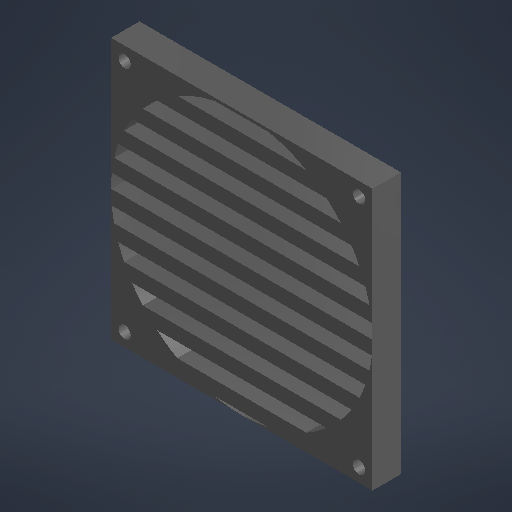
# Autodesk Inventor part: PlaqueProtectionVentilo
Saved by Autodesk Inventor 2026.2 (Build 302298010, 298A)
## iProperties
Part Number: PlaqueProtectionVentilo
Material: Générique
Document SubType Name: Modélisation
Designer: quent
Appearance: Par défaut
Author: quent
Autodesk Inventor part; units mm, degrees
ref_plane "Plan YZ" through (0, 0, 0) normal (1, 0, 0) x (0, 1, 0)
ref_plane "Plan XZ" through (0, 0, 0) normal (0, 1, 0) x (-1, 0, 0)
ref_plane "Plan XY" through (0, 0, 0) normal (0, 0, 1) x (1, 0, 0)
sketch "Esquisse1" plane through (0, 0, 0) normal (0, 0, 1) x (1, 0, 0)
  line L0 (-45.1239, -31.1354) -> (-45.1239, 20.8646)
  circle A0 centre (-40.3739, -46.3854) radius 2.2
  circle A1 centre (-40.3739, 36.1146) radius 2.2
  line L1 (-25.1239, 40.8646) -> (-45.1239, 20.8646)
  line L2 (-45.1239, -31.1354) -> (-25.1239, -51.1354)
  line L3 (26.8761, -51.1354) -> (-25.1239, -51.1354)
  line L4 (-25.1239, 40.8646) -> (26.8761, 40.8646)
  circle A2 centre (42.1261, -46.3854) radius 2.2
  line L5 (26.8761, -51.1354) -> (46.8761, -31.1354)
  line L6 (46.8761, 20.8646) -> (46.8761, -31.1354)
  line L7 (46.8761, 40.8646) -> (-45.1239, -51.1354) construction
  line L8 (-45.1239, 40.8646) -> (46.8761, -51.1354) construction
  circle A3 centre (42.1261, 36.1146) radius 2.2
  line L9 (46.8761, 20.8646) -> (26.8761, 40.8646)
  line L10 (-45.1239, 40.8646) -> (46.8761, 40.8646)
  line L11 (46.8761, 40.8646) -> (46.8761, -51.1354)
  line L12 (46.8761, -51.1354) -> (-45.1239, -51.1354)
  line L13 (-45.1239, -51.1354) -> (-45.1239, 40.8646)
  circle A4 centre (0.8761, -5.1354) radius 46
  line L14 (-45.1239, 39.8646) -> (46.8761, 39.8646)
  line L15 (46.8761, 39.8646) -> (46.8761, 34.8646)
  line L16 (46.8761, 34.8646) -> (-45.1239, 34.8646)
  line L17 (-45.1239, 34.8646) -> (-45.1239, 39.8646)
  line L18 (-28.9735, 29.8646) -> (30.7257, 29.8646)
  line L19 (-33.9951, 24.8646) -> (35.7473, 24.8646)
  line L20 (-37.7374, 19.8646) -> (39.4896, 19.8646)
  line L21 (-40.5485, 14.8646) -> (42.3007, 14.8646)
  line L22 (-37.7374, 19.8646) -> (39.4896, 19.8646)
  line L23 (-42.6095, 9.8646) -> (44.3617, 9.8646)
  line L24 (-44.0238, 4.8646) -> (45.776, 4.8646)
  line L25 (-45.1239, -5.1354) -> (46.8761, -5.1354)
  line L26 (-44.8514, -0.1354) -> (46.6035, -0.1354)
  line L27 (-44.8514, -10.1354) -> (46.6035, -10.1354)
  line L28 (-44.0238, -15.1354) -> (45.776, -15.1354)
  line L29 (-42.6095, -20.1354) -> (44.3617, -20.1354)
  line L30 (-40.5485, -25.1354) -> (42.3007, -25.1354)
  line L31 (-37.7374, -30.1354) -> (39.4896, -30.1354)
  line L32 (-33.9951, -35.1354) -> (35.7473, -35.1354)
  line L33 (-28.9735, -40.1354) -> (30.7257, -40.1354)
  line L34 (-21.8395, -45.1354) -> (23.5917, -45.1354)
  line L35 (-8.6633, -50.1354) -> (10.4155, -50.1354)
  point P0 (0, 0)
  point P1 (-0.1239, 48.3646)
  point P2 (-45.1239, -5.1354)
  point P3 (-45.1239, -5.1354)
  point P4 (0.8761, -51.1354)
  point P5 (46.8761, -5.1354)
  point P6 (46.8761, -5.1354)
  point P7 (10.4155, 39.8646)
  point P8 (23.5917, 34.8646)
  point P9 (-21.8395, 34.8646)
  point P10 (-8.6633, 39.8646)
  dimension "d0" = 92
  dimension "d1" = 92
  dimension "d2" = 20
  dimension "d3" = 20
  dimension "d4" = 20
  dimension "d5" = 20
  dimension "d6" = 20
  dimension "d7" = 20
  dimension "d8" = 20
  dimension "d9" = 20
  dimension "d10" = 4.4
  dimension "d11" = 4.4
  dimension "d12" = 4.4
  dimension "d13" = 4.4
  dimension "d14" = 4.75
  dimension "d15" = 4.75
  dimension "d16" = 5
  dimension "d17" = 5
  dimension "d18" = 5
  dimension "d19" = 5
  dimension "d20" = 5
  dimension "d21" = 5
  dimension "d22" = 5
  dimension "d23" = 5
  dimension "d25" = 5
  dimension "d26" = 5
  dimension "d27" = 5
  dimension "d28" = 5
  dimension "d29" = 5
  dimension "d30" = 5
  dimension "d31" = 5
  dimension "d32" = 5
  dimension "d33" = 5
  dimension "d34" = 5
  dimension "d35" = 5
  constraints: 72 end point, 21 point on line, 18 parallel, 4 centre point, 4 horizontal, 4 midpoint, 3 perpendicular, 1 coincident, 38 other
  measures "d0" distance of L8.end L7.end
  measures "d1" distance of L7.start L8.end
  measures "d2" distance of L1.start point (-45.124, 40.865)
  measures "d3" distance of L1.end point (-45.124, 40.865)
  measures "d4" distance of L2.start point (-45.124, -51.135)
  measures "d5" distance of L2.end point (-45.124, -51.135)
  measures "d6" distance of L5.start point (46.876, -51.135)
  measures "d7" distance of L5.end point (46.876, -51.135)
  measures "d8" distance of L9.start point (46.876, 40.865)
  measures "d9" distance of L9.end point (46.876, 40.865)
  measures "d10" diameter of A1
  measures "d11" diameter of A3
  measures "d12" diameter of A2
  measures "d13" diameter of A0
  measures "d14" horizontal distance of L8.start A1.centre
  measures "d15" horizontal distance of L8.start A1.centre
  measures "d16" distance between parallel lines of L16 L14
  measures "d17" distance between parallel lines of L18 L16
  measures "d18" distance between parallel lines of L19 L18
  measures "d19" distance between parallel lines of L20 L19
  measures "d20" distance between parallel lines of L21 L20
  measures "d21" distance between parallel lines of L21 L22
  measures "d22" distance between parallel lines of L23 L21
  measures "d23" distance between parallel lines of L24 L23
  measures "d25" distance between parallel lines of L26 L24
  measures "d26" distance between parallel lines of L25 L26
  measures "d27" distance between parallel lines of L27 L25
  measures "d28" distance between parallel lines of L28 L27
  measures "d29" distance between parallel lines of L29 L28
  measures "d30" distance between parallel lines of L30 L29
  measures "d31" distance between parallel lines of L31 L30
  measures "d32" distance between parallel lines of L32 L31
  measures "d33" distance between parallel lines of L33 L32
  measures "d34" distance between parallel lines of L34 L33
  measures "d35" distance between parallel lines of L35 L34
extrude "Extrusion1" add sketch "Esquisse1" along normal blind 10 contours L0 A4 L3 L2 | L2 L12 L13 | L0 L1 L16 A4 | L25 A4 L27 | L13 L16 A1 L1 | A4 L24 L26 | A4 L16 L9 L6 | L6 L5 L3 A4 | L16 A1 L13 L14 L1 | L1 L14 A4 L16 | L28 A4 L29 | L9 L16 A3 L11 | L11 L12 L5 | A4 L34 L35 | L14 L13 L10 L1 | L1 L4 A4 L14 | L16 A4 L18 | A4 L21 L23 | L16 A4 L14 L9 | L9 L14 L11 L16 A3 | A4 L14 | L30 A4 L31 | L14 A4 L4 L9 | L9 L10 L11 L14 | A4 L32 L33 | L19 A4 L20
equation "\"d3\" = d2"
equation "\"d4\" = d2"
equation "\"d5\" = d4"
equation "\"d6\" = d2"
equation "\"d7\" = d6"
equation "\"d8\" = d2"
equation "\"d9\" = d8"
